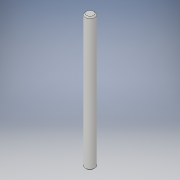
# Autodesk Inventor part: ABI_Arretierstift
Saved by Autodesk Inventor 2018 (Build 220112000, 112)
## iProperties
Created: 2019-11-22
Part Number: ABI_Arretierstift
Material: Generisch
Document SubType Name: Modeling
Designer: Dubsky
Density: 1 g/cm^3
Appearance: Vorgabe
Author: Dubsky
Autodesk Inventor part; units mm, degrees
ref_plane "YZ Plane" through (0, 0, 0) normal (1, 0, 0) x (0, 1, 0)
ref_plane "XZ Plane" through (0, 0, 0) normal (0, 1, 0) x (-1, 0, 0)
ref_plane "XY Plane" through (0, 0, 0) normal (0, 0, 1) x (1, 0, 0)
sketch "Skizze1" plane through (0, 0, 0) normal (0, 0, 1) x (1, 0, 0)
  circle A0 centre (0, 0) radius 2
  dimension "Durchmesser" = 4
  constraints: 1 centre point, 1 coincident
  measures "Durchmesser" diameter of A0
extrude "Extrusion1" add sketch "Skizze1" along normal blind 55
chamfer "Fase1" distance 0.5 angle 45 1 edges at (-2, 0, 0) measured on face at (0.6473, -0.1595, 0)
chamfer "Fase2" distance 0.5 angle 45 1 edges at (-2, 0, 55) measured on face at (1.9935, -0.1609, 36.8333)
